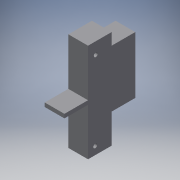
# Autodesk Inventor part: 00_Microlinearmotor
Saved by Autodesk Inventor 2019.4 (Build 234330000, 330)
## iProperties
Created: 2021-09-28
Part Number: 00_Microlinearmotor
Material: Generic
Document SubType Name: Modeling
Designer: diederichbenedict
Density: 1 g/cm^3
Appearance: Default
Author: diederichbenedict
Autodesk Inventor part; units mm, degrees
ref_plane "YZ Plane" through (0, 0, 0) normal (1, 0, 0) x (0, 1, 0)
ref_plane "XZ Plane" through (0, 0, 0) normal (0, 1, 0) x (-1, 0, 0)
ref_plane "XY Plane" through (0, 0, 0) normal (0, 0, 1) x (1, 0, 0)
sketch "Sketch1" plane through (0, 0, 0) normal (1, 0, 0) x (0, 1, 0)
  line L0 (-5.0178, 2.5025) -> (19.9822, 2.5025)
  line L1 (19.9822, 2.5025) -> (19.9822, -3.4975)
  line L2 (19.9822, -3.4975) -> (-5.0178, -3.4975)
  line L3 (-5.0178, -3.4975) -> (-5.0178, 2.5025)
  circle A0 centre (-3.0178, 0.668) radius 0.5
  circle A1 centre (16.9818, 0.5397) radius 0.5
  line L4 (16.9822, -3.4975) -> (2.4822, -3.4975)
  line L5 (2.4822, -3.4975) -> (2.4822, -9.4975)
  line L6 (2.4822, -9.4975) -> (16.9822, -9.4975)
  line L7 (16.9822, -9.4975) -> (16.9822, -3.4975)
  line L8 (7.9822, 2.5025) -> (6.9822, 2.5025)
  line L9 (6.9822, 2.5025) -> (6.9822, 8.5025)
  line L10 (6.9822, 8.5025) -> (7.9822, 8.5025)
  line L11 (7.9822, 8.5025) -> (7.9822, 2.5025)
  point P0 (0, 0)
  dimension "d0" = 25
  dimension "d1" = 6
  dimension "d2" = 1
  dimension "d3" = 1
  dimension "d4" = 20
  dimension "d5" = 14.5
  dimension "d6" = 6
  dimension "d7" = 7.5
  dimension "d8" = 1
  dimension "d9" = 6
  dimension "d10" = 10
  dimension "d13" = 2
  constraints: 24 end point, 6 parallel, 3 horizontal, 3 perpendicular, 2 centre point, 2 point on line
  measures "d0" distance of L1.end L2.end
  measures "d1" distance of L0.end L1.end
  measures "d2" diameter of A0
  measures "d3" diameter of A1
  measures "d4" distance of A0.centre A1.centre
  measures "d5" distance of L6.end L5.end
  measures "d6" distance of L5.end L4.end
  measures "d7" distance between parallel lines of L3 L5
  measures "d8" distance of L9.end L10.end
  measures "d9" distance of L8.end L9.end
  measures "d10" distance from line of L9 A0.centre
  measures "d13" distance from line of A0.centre L3
extrude "Extrusion1" add sketch "Sketch1" along normal blind 5
body "Solid1"
